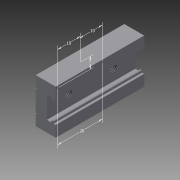
# Autodesk Inventor part: Karetka
Saved by Autodesk Inventor 2015 (Build 190159000, 159)
## iProperties
Created: 2016-04-08
Part Number: Karetka
Material: Generic
Document SubType Name: Modeling
Designer: Andreas
Density: 1 g/cm^3
Appearance: Default
Author: Andreas
Autodesk Inventor part; units mm, degrees
ref_plane "YZ Plane" through (0, 0, 0) normal (1, 0, 0) x (0, 1, 0)
ref_plane "XZ Plane" through (0, 0, 0) normal (0, 1, 0) x (-1, 0, 0)
ref_plane "XY Plane" through (0, 0, 0) normal (0, 0, 1) x (1, 0, 0)
sketch "Sketch1" plane through (0, 0, 0) normal (0, 1, 0) x (-1, 0, 0)
  line L0 (0, 0) -> (0, 5)
  line L1 (0, 5) -> (9, 5)
  line L2 (9, 5) -> (9, -15)
  line L3 (9, -15) -> (0, -15)
  line L4 (0, -15) -> (0, -10)
  line L5 (0, -10) -> (4, -10)
  line L6 (4, -10) -> (4, 0)
  line L7 (4, 0) -> (0, 0)
  dimension "d0" = 5
  dimension "d1" = 9
  dimension "d2" = 20
  dimension "d3" = 9
  dimension "d4" = 5
  dimension "d5" = 4
  dimension "d6" = 10
  constraints: 16 end point, 5 perpendicular, 2 vertical
  measures "d0" distance of L0.start L0.end
  measures "d1" distance of L0.end L1.end
  measures "d2" distance of L1.end L2.end
  measures "d3" distance of L2.end L3.end
  measures "d4" distance of L3.end L4.end
  measures "d5" distance of L4.end L5.end
  measures "d6" distance of L5.end L6.end
extrude "Extrusion1" add sketch "Sketch1" along normal blind 40
sketch "Sketch2" plane through (-9, 0, -15) normal (-1, 0, 0) x (0, 0, 1)
  line L0 (5, 0) -> (5, 40) projected
  line L1 (15, 0) -> (15, 40) projected
  point P0 (15, 20)
  point P1 (10, 10)
  point P2 (10, 30)
  dimension "d9" = 5
  dimension "d10" = 10
  dimension "d11" = 20
  dimension "d12" = 10
  constraints: 1 midpoint
  measures "d9" horizontal distance of point (15, 20) point (10, 10)
  measures "d10" vertical distance of point (15, 20) point (10, 10)
  measures "d11" distance of point (10, 30) point (10, 10)
  measures "d12" vertical distance of point (10, 30) point (15, 20)
sketch "Sketch4" plane through (-4, 0, 0) normal (1, 0, 0) x (0, 0, -1)
  point P0 (5, 30)
  point P1 (5, 10)
hole "Hole2" at (-4, 30, -5) at (-4, 10, -5) direction (-1, 0, 0) diameter 3.4 depth 5
thread "Thread3" size "M4x0.7" class "6H" standard "ANSI Metric M Profile" full length
thread "Thread4" size "M3.5x0.6" class "6H" standard "ANSI Metric M Profile" full length
sketch "Sketch5" plane through (0, 0, 0) normal (0, -1, 0) x (1, 0, 0)
  line L0 (-1, -10) -> (-1, -9.5)
  line L1 (-1.5, -9) -> (-1.5, -9)
  line L2 (-2, -9.5) -> (-2, -10)
  line L3 (-2, -10) -> (-1, -10)
  line L4 (-1, -0.5) -> (-1, 0)
  line L5 (-1, 0) -> (-2, 0)
  line L6 (-2, 0) -> (-2, -0.5)
  line L7 (-1.5, -1) -> (-1.5, -1)
  arc A0 (-1.5, -9) -> (-2, -9.5) centre (-1.5, -9.5) ccw
  arc A1 (-1, -9.5) -> (-1.5, -9) centre (-1.5, -9.5) ccw
  arc A2 (-2, -0.5) -> (-1.5, -1) centre (-1.5, -0.5) ccw
  arc A3 (-1.5, -1) -> (-1, -0.5) centre (-1.5, -0.5) ccw
  point P0 (0, 0)
  point P1 (-1, -9)
  point P2 (-2, -9)
  point P3 (-1, -1)
  point P4 (-2, -1)
  point P5 (-1.5, 0)
  point P6 (-1.5, -10)
  point P7 (0, -10)
  dimension "d35" = 1
  dimension "d36" = 1
  dimension "d37" = 1
  dimension "d38" = 1
  dimension "d39" = 1
  dimension "d40" = 1
  dimension "d41" = 0.5
  dimension "d42" = 1
  dimension "d43" = 1
  constraints: 16 end point, 10 point on line, 8 point on circle, 8 tangent, 4 centre point, 3 equal radius, 3 perpendicular, 2 horizontal alignment, 2 midpoint, 1 horizontal, 1 vertical
  measures "d35" distance of L0.start point (-1, -9)
  measures "d36" distance of point (-1, -9) point (-2, -9)
  measures "d37" distance of point (-2, -9) L2.end
  measures "d38" distance of point (-1, -1) L4.end
  measures "d39" distance of L4.end L5.end
  measures "d40" distance of L5.end point (-2, -1)
  measures "d41" radius of A0
  measures "d42" distance from line of point (0, -10) L0
  measures "d43" horizontal distance of point (0, 0) L4.start
extrude "Extrusion2" add sketch "Sketch5" against normal blind 40
body "Solid1"
